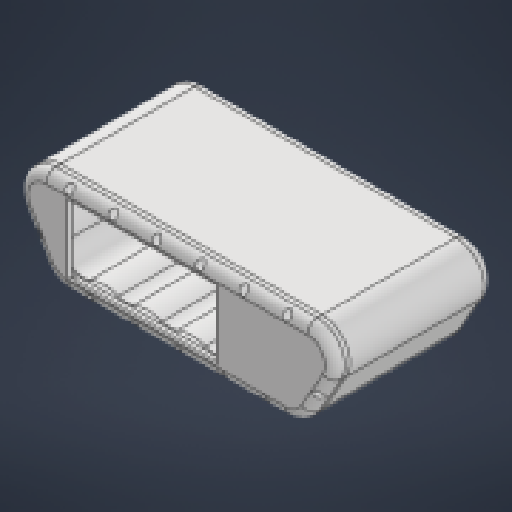
# Autodesk Inventor part: frame
Saved by Autodesk Inventor 2024 (Build 280153000, 153)
## iProperties
Created: 2024-05-04
Part Number: frame
Material: Generic
Document SubType Name: Modeling
Designer: markm
Density: 1 g/cm^3
Appearance: Default
Author: markm
Autodesk Inventor part; units mm, degrees
ref_plane "YZ Plane" through (0, 0, 0) normal (1, 0, 0) x (0, 1, 0)
ref_plane "XZ Plane" through (0, 0, 0) normal (0, 1, 0) x (-1, 0, 0)
ref_plane "XY Plane" through (0, 0, 0) normal (0, 0, 1) x (1, 0, 0)
sketch "Sketch1" plane through (0, 0, 0) normal (0, 0, 1) x (1, 0, 0)
  line L0 (0, -30.8093) -> (0, 30.8093) construction
  line L1 (78.1244, 2.5263) -> (67.1244, -16.5263)
  line L2 (55, -23.5263) -> (-55, -23.5263)
  line L3 (-67.1244, -16.5263) -> (-78.1244, 2.5263)
  arc A0 (-66, 23.5263) -> (-78.1244, 2.5263) centre (-66, 9.5263) ccw
  arc A1 (78.1244, 2.5263) -> (66, 23.5263) centre (66, 9.5263) ccw
  line L4 (-66, 9.5263) -> (-55, -9.5263) construction
  line L5 (-55, -9.5263) -> (55, -9.5263) construction
  line L6 (55, -9.5263) -> (66, 9.5263) construction
  line L7 (66, 9.5263) -> (-66, 9.5263) construction
  circle A2 centre (-66, 9.5263) radius 11
  circle A3 centre (-55, -9.5263) radius 11
  circle A4 centre (66, 9.5263) radius 11
  line L8 (-60.5, 0) -> (60.5, 0) construction
  circle A5 centre (-44, 9.5263) radius 11
  circle A6 centre (-33, -9.5263) radius 11
  circle A7 centre (-22, 9.5263) radius 11
  circle A8 centre (-11, -9.5263) radius 11
  circle A9 centre (0, 9.5263) radius 11
  circle A10 centre (11, -9.5263) radius 11
  circle A11 centre (22, 9.5263) radius 11
  circle A12 centre (33, -9.5263) radius 11
  circle A13 centre (44, 9.5263) radius 11
  circle A14 centre (55, -9.5263) radius 11
  arc A15 (-67.1244, -16.5263) -> (-55, -23.5263) centre (-55, -9.5263) ccw
  arc A16 (55, -23.5263) -> (67.1244, -16.5263) centre (55, -9.5263) ccw
  line L9 (-66, 23.5263) -> (66, 23.5263)
  arc A17 (75.9593, 3.7763) -> (66, 21.0263) centre (66, 9.5263) ccw construction
  line L10 (75.9593, 3.7763) -> (64.9593, -15.2763) construction
  arc A18 (55, -21.0263) -> (64.9593, -15.2763) centre (55, -9.5263) ccw construction
  line L11 (55, -21.0263) -> (-55, -21.0263) construction
  arc A19 (-64.9593, -15.2763) -> (-55, -21.0263) centre (-55, -9.5263) ccw construction
  line L12 (-64.9593, -15.2763) -> (-75.9593, 3.7763) construction
  arc A20 (-66, 21.0263) -> (-75.9593, 3.7763) centre (-66, 9.5263) ccw construction
  line L13 (-66, 21.0263) -> (66, 21.0263) construction
  arc A21 (72.9412, 0.9928) -> (65.8608, -11.2708) centre (85.4801, -14.4223) ccw
  line L14 (66, 9.5263) -> (33, -9.5263) construction
  line L15 (55, -9.5263) -> (44, 9.5263) construction
  arc A22 (47.9196, 19.8043) -> (62.0804, 19.8043) centre (55, 38.3708) ccw
  arc A23 (51.0804, -19.8043) -> (36.9196, -19.8043) centre (44, -38.3708) ccw
  line L16 (85.4801, -14.4223) -> (70.4593, -5.75) construction
  line L17 (55, 18.5) -> (55, 21.0263) construction
  line L18 (44, -18.5) -> (44, -21.0263) construction
  arc A24 (25.9196, 19.8043) -> (40.0804, 19.8043) centre (33, 38.3708) ccw
  line L19 (33, 18.5) -> (33, 21.0263) construction
  line L20 (22, -18.5) -> (22, -21.0263) construction
  arc A25 (29.0804, -19.8043) -> (14.9196, -19.8043) centre (22, -38.3708) ccw
  arc A26 (3.9196, 19.8043) -> (18.0804, 19.8043) centre (11, 38.3708) ccw
  line L21 (11, 18.5) -> (11, 21.0263) construction
  line L22 (0, -18.5) -> (0, -21.0263) construction
  arc A27 (7.0804, -19.8043) -> (-7.0804, -19.8043) centre (0, -38.3708) ccw
  arc A28 (-18.0804, 19.8043) -> (-3.9196, 19.8043) centre (-11, 38.3708) ccw
  line L23 (-11, 18.5) -> (-11, 21.0263) construction
  line L24 (-22, -18.5) -> (-22, -21.0263) construction
  arc A29 (-14.9196, -19.8043) -> (-29.0804, -19.8043) centre (-22, -38.3708) ccw
  arc A30 (-40.0804, 19.8043) -> (-25.9196, 19.8043) centre (-33, 38.3708) ccw
  line L25 (-33, 18.5) -> (-33, 21.0263) construction
  line L26 (-44, -18.5) -> (-44, -21.0263) construction
  arc A31 (-36.9196, -19.8043) -> (-51.0804, -19.8043) centre (-44, -38.3708) ccw
  arc A32 (-65.8608, -11.2708) -> (-72.9412, 0.9928) centre (-85.4801, -14.4223) ccw
  arc A33 (-62.0804, 19.8043) -> (-47.9196, 19.8043) centre (-55, 38.3708) ccw
  line L27 (-85.4801, -14.4223) -> (-70.4593, -5.75) construction
  line L28 (-55, 18.5) -> (-55, 21.0263) construction
  point P0 (0, 0)
  point P1 (0, 0)
  point P2 (44, -9.5263)
  point P3 (22, -9.5263)
  point P4 (0, -9.5263)
  point P5 (-22, -9.5263)
  point P6 (-44, -9.5263)
  point P7 (-60.5, 0)
  point P8 (-55, 9.5263)
  point P9 (-33, 9.5263)
  point P10 (-11, 9.5263)
  point P11 (11, 9.5263)
  point P12 (33, 9.5263)
  point P13 (55, 9.5263)
  point P14 (60.5, 0)
  point P15 (80, 9.5263)
  point P16 (47.9196, 19.8043)
  point P17 (62.0804, 19.8043)
  point P18 (51.0804, -19.8043)
  point P19 (36.9196, -19.8043)
  point P20 (-49.5, 0)
  point P21 (-38.5, 0)
  point P22 (-27.5, 0)
  point P23 (-16.5, 0)
  point P24 (-5.5, 0)
  point P25 (5.5, 0)
  point P26 (16.5, 0)
  point P27 (27.5, 0)
  point P28 (38.5, 0)
  point P29 (49.5, 0)
  point P30 (-62.0804, 19.8043)
  point P31 (-47.9196, 19.8043)
  point P32 (-40.0804, 19.8043)
  point P33 (-25.9196, 19.8043)
  point P34 (-18.0804, 19.8043)
  point P35 (-3.9196, 19.8043)
  point P36 (3.9196, 19.8043)
  point P37 (18.0804, 19.8043)
  point P38 (25.9196, 19.8043)
  point P39 (40.0804, 19.8043)
  point P40 (29.0804, -19.8043)
  point P41 (14.9196, -19.8043)
  point P42 (7.0804, -19.8043)
  point P43 (-7.0804, -19.8043)
  point P44 (-14.9196, -19.8043)
  point P45 (-29.0804, -19.8043)
  point P46 (-36.9196, -19.8043)
  point P47 (-51.0804, -19.8043)
  point P48 (-65.8608, -11.2708)
  point P49 (-72.9412, 0.9928)
  dimension "d70" = 22
  dimension "d73" = 22
  dimension "d106" = 14
  dimension "d122" = 14
  dimension "d174" = 2.5
  dimension "d182" = 37
  dimension "d185" = 22
  constraints: 59 end point, 45 point on circle, 32 centre point, 15 symmetric about line, 7 tangent, 5 coincident, 5 horizontal, 5 midpoint, 3 equal radius, 2 perpendicular, 2 point on line, 1 parallel, 101 other
  measures "d70" diameter of A2
  measures "d73" distance of A2.centre A5.centre
  measures "d106" radius of A16
  measures "d122" distance between parallel lines of L2 L5
  measures "d174" distance between parallel lines of L9 L13
  measures "d182" vertical distance of L18.start L17.start
  measures "d185" distance of A22.centre A24.centre
extrude "Extrusion1" add sketch "Sketch1" along normal mid plane 65
sketch "Sketch16" plane through (0, 0, -32.5) normal (0, 0, -1) x (-1, 0, 0)
  line L0 (67.1244, -16.5263) -> (78.1244, 2.5263) projected
  arc A0 (78.1244, 2.5263) -> (66, 23.5263) centre (66, 9.5263) ccw projected
  line L1 (66, 23.5263) -> (-66, 23.5263) projected
  arc A1 (-66, 23.5263) -> (-78.1244, 2.5263) centre (-66, 9.5263) ccw projected
  line L2 (-78.1244, 2.5263) -> (-67.1244, -16.5263) projected
  arc A2 (-67.1244, -16.5263) -> (-55, -23.5263) centre (-55, -9.5263) ccw projected
  line L3 (-55, -23.5263) -> (55, -23.5263) projected
  arc A3 (55, -23.5263) -> (67.1244, -16.5263) centre (55, -9.5263) ccw projected
  arc A4 (47.9196, 19.8043) -> (62.0804, 19.8043) centre (55, 38.3708) ccw projected
  arc A5 (72.9412, 0.9928) -> (62.0804, 19.8043) centre (66, 9.5263) ccw projected
  arc A6 (72.9412, 0.9928) -> (65.8608, -11.2708) centre (85.4801, -14.4223) ccw projected
  arc A7 (51.0804, -19.8043) -> (65.8608, -11.2708) centre (55, -9.5263) ccw projected
  arc A8 (51.0804, -19.8043) -> (36.9196, -19.8043) centre (44, -38.3708) ccw projected
  arc A9 (29.0804, -19.8043) -> (36.9196, -19.8043) centre (33, -9.5263) ccw projected
  arc A10 (29.0804, -19.8043) -> (14.9196, -19.8043) centre (22, -38.3708) ccw projected
  arc A11 (7.0804, -19.8043) -> (14.9196, -19.8043) centre (11, -9.5263) ccw projected
  arc A12 (7.0804, -19.8043) -> (-7.0804, -19.8043) centre (0, -38.3708) ccw projected
  arc A13 (-14.9196, -19.8043) -> (-7.0804, -19.8043) centre (-11, -9.5263) ccw projected
  arc A14 (-14.9196, -19.8043) -> (-29.0804, -19.8043) centre (-22, -38.3708) ccw projected
  arc A15 (-36.9196, -19.8043) -> (-29.0804, -19.8043) centre (-33, -9.5263) ccw projected
  arc A16 (-36.9196, -19.8043) -> (-51.0804, -19.8043) centre (-44, -38.3708) ccw projected
  arc A17 (-65.8608, -11.2708) -> (-51.0804, -19.8043) centre (-55, -9.5263) ccw projected
  arc A18 (-65.8608, -11.2708) -> (-72.9412, 0.9928) centre (-85.4801, -14.4223) ccw projected
  arc A19 (-62.0804, 19.8043) -> (-72.9412, 0.9928) centre (-66, 9.5263) ccw projected
  arc A20 (-62.0804, 19.8043) -> (-47.9196, 19.8043) centre (-55, 38.3708) ccw projected
  arc A21 (-40.0804, 19.8043) -> (-47.9196, 19.8043) centre (-44, 9.5263) ccw projected
  arc A22 (-40.0804, 19.8043) -> (-25.9196, 19.8043) centre (-33, 38.3708) ccw projected
  arc A23 (-18.0804, 19.8043) -> (-25.9196, 19.8043) centre (-22, 9.5263) ccw projected
  arc A24 (-18.0804, 19.8043) -> (-3.9196, 19.8043) centre (-11, 38.3708) ccw projected
  arc A25 (3.9196, 19.8043) -> (-3.9196, 19.8043) centre (0, 9.5263) ccw projected
  arc A26 (3.9196, 19.8043) -> (18.0804, 19.8043) centre (11, 38.3708) ccw projected
  arc A27 (25.9196, 19.8043) -> (18.0804, 19.8043) centre (22, 9.5263) ccw projected
  arc A28 (25.9196, 19.8043) -> (40.0804, 19.8043) centre (33, 38.3708) ccw projected
  arc A29 (47.9196, 19.8043) -> (40.0804, 19.8043) centre (44, 9.5263) ccw projected
  line L4 (-66, 18.5) -> (66, 18.5)
  arc A30 (73.7715, 5.0394) -> (66, 18.5) centre (66, 9.5263) ccw
  line L5 (73.7715, 5.0394) -> (62.7715, -14.0131)
  arc A31 (55, -18.5) -> (62.7715, -14.0131) centre (55, -9.5263) ccw
  line L6 (55, -18.5) -> (-55, -18.5)
  arc A32 (-62.7715, -14.0131) -> (-55, -18.5) centre (-55, -9.5263) ccw
  line L7 (-62.7715, -14.0131) -> (-73.7715, 5.0394)
  arc A33 (-66, 18.5) -> (-73.7715, 5.0394) centre (-66, 9.5263) ccw
  point P0 (0, 0)
  constraints: 8 end point, 8 point on circle, 4 centre point, 1 tangent, 7 other
extrude "Extrusion14" add sketch "Sketch16" along normal blind 7.5 contours A3 L3 A2 L2 A1 L1 A0 L0 | A4 L4 A28 A29 | L4 A30 L5 A31 L6 A32 L7 A33 | A4 A5 A6 L5 A30 L4 | L4 A26 A27 A28 | L4 A24 A25 A26 | A6 A7 A8 L6 A31 L5 | L4 A22 A23 A24 | L4 A20 A21 A22 | L4 A33 L7 A18 A19 A20 | A8 A9 A10 L6 | A10 A11 A12 L6 | A12 A13 A14 L6 | L7 A32 L6 A16 A17 A18 | A14 A15 A16 L6
extrude "Extrusion16" cut sketch "Sketch16" along normal blind 2.5 contours A4 L4 A28 A29 | L4 A30 L5 A31 L6 A32 L7 A33 | A4 A5 A6 L5 A30 L4 | L4 A26 A27 A28 | L4 A24 A25 A26 | A6 A7 A8 L6 A31 L5 | L4 A22 A23 A24 | L4 A20 A21 A22 | L4 A33 L7 A18 A19 A20 | A8 A9 A10 L6 | A10 A11 A12 L6 | A12 A13 A14 L6 | L7 A32 L6 A16 A17 A18 | A14 A15 A16 L6
extrude "Extrusion15" cut sketch "Sketch16" along normal blind 5 contours L4 A30 L5 A31 L6 A32 L7 A33
fillet "Fillet6" radius 5 8 edges at (78.1244, 16.5263, -40) (72.6244, -7, -40) (62, -21.6506, -40) (0, -23.5263, -40) (-62, -21.6506, -40) (-72.6244, -7, -40) (-78.1244, 16.5263, -40) (0, 23.5263, -40)
sketch "Sketch20" plane through (0, 0, 32.5) normal (0, 0, 1) x (1, 0, 0)
  line L0 (-78.1244, 2.5263) -> (-67.1244, -16.5263) projected
  arc A0 (-67.1244, -16.5263) -> (-55, -23.5263) centre (-55, -9.5263) ccw projected
  line L1 (-55, -23.5263) -> (55, -23.5263) projected
  arc A1 (55, -23.5263) -> (67.1244, -16.5263) centre (55, -9.5263) ccw projected
  line L2 (67.1244, -16.5263) -> (78.1244, 2.5263) projected
  arc A2 (78.1244, 2.5263) -> (66, 23.5263) centre (66, 9.5263) ccw projected
  line L3 (66, 23.5263) -> (-66, 23.5263) projected
  arc A3 (-66, 23.5263) -> (-78.1244, 2.5263) centre (-66, 9.5263) ccw projected
  arc A4 (-62.0804, 19.8043) -> (-47.9196, 19.8043) centre (-55, 38.3708) ccw projected
  arc A5 (-40.0804, 19.8043) -> (-47.9196, 19.8043) centre (-44, 9.5263) ccw projected
  arc A6 (-40.0804, 19.8043) -> (-25.9196, 19.8043) centre (-33, 38.3708) ccw projected
  arc A7 (-18.0804, 19.8043) -> (-25.9196, 19.8043) centre (-22, 9.5263) ccw projected
  arc A8 (-18.0804, 19.8043) -> (-3.9196, 19.8043) centre (-11, 38.3708) ccw projected
  arc A9 (3.9196, 19.8043) -> (-3.9196, 19.8043) centre (0, 9.5263) ccw projected
  arc A10 (3.9196, 19.8043) -> (18.0804, 19.8043) centre (11, 38.3708) ccw projected
  arc A11 (25.9196, 19.8043) -> (18.0804, 19.8043) centre (22, 9.5263) ccw projected
  arc A12 (25.9196, 19.8043) -> (40.0804, 19.8043) centre (33, 38.3708) ccw projected
  arc A13 (47.9196, 19.8043) -> (40.0804, 19.8043) centre (44, 9.5263) ccw projected
  arc A14 (47.9196, 19.8043) -> (62.0804, 19.8043) centre (55, 38.3708) ccw projected
  arc A15 (72.9412, 0.9928) -> (62.0804, 19.8043) centre (66, 9.5263) ccw projected
  arc A16 (72.9412, 0.9928) -> (65.8608, -11.2708) centre (85.4801, -14.4223) ccw projected
  arc A17 (51.0804, -19.8043) -> (65.8608, -11.2708) centre (55, -9.5263) ccw projected
  arc A18 (51.0804, -19.8043) -> (36.9196, -19.8043) centre (44, -38.3708) ccw projected
  arc A19 (29.0804, -19.8043) -> (36.9196, -19.8043) centre (33, -9.5263) ccw projected
  arc A20 (29.0804, -19.8043) -> (14.9196, -19.8043) centre (22, -38.3708) ccw projected
  arc A21 (7.0804, -19.8043) -> (14.9196, -19.8043) centre (11, -9.5263) ccw projected
  arc A22 (7.0804, -19.8043) -> (-7.0804, -19.8043) centre (0, -38.3708) ccw projected
  arc A23 (-14.9196, -19.8043) -> (-7.0804, -19.8043) centre (-11, -9.5263) ccw projected
  arc A24 (-14.9196, -19.8043) -> (-29.0804, -19.8043) centre (-22, -38.3708) ccw projected
  arc A25 (-36.9196, -19.8043) -> (-29.0804, -19.8043) centre (-33, -9.5263) ccw projected
  arc A26 (-36.9196, -19.8043) -> (-51.0804, -19.8043) centre (-44, -38.3708) ccw projected
  arc A27 (-65.8608, -11.2708) -> (-51.0804, -19.8043) centre (-55, -9.5263) ccw projected
  arc A28 (-65.8608, -11.2708) -> (-72.9412, 0.9928) centre (-85.4801, -14.4223) ccw projected
  arc A29 (-62.0804, 19.8043) -> (-72.9412, 0.9928) centre (-66, 9.5263) ccw projected
  line L4 (-66, 18.5) -> (66, 18.5)
  arc A30 (73.7715, 5.0394) -> (66, 18.5) centre (66, 9.5263) ccw
  line L5 (73.7715, 5.0394) -> (62.7715, -14.0131)
  arc A31 (55, -18.5) -> (62.7715, -14.0131) centre (55, -9.5263) ccw
  line L6 (55, -18.5) -> (-55, -18.5)
  arc A32 (-62.7715, -14.0131) -> (-55, -18.5) centre (-55, -9.5263) ccw
  line L7 (-62.7715, -14.0131) -> (-73.7715, 5.0394)
  arc A33 (-66, 18.5) -> (-73.7715, 5.0394) centre (-66, 9.5263) ccw
  arc A34 (-65.8608, -11.2708) -> (-72.9412, 0.9928) centre (-85.4801, -14.4223) ccw projected
  point P0 (0, 0)
  constraints: 8 end point, 8 point on circle, 4 centre point, 1 tangent, 7 other
extrude "Extrusion17" add sketch "Sketch20" along normal blind 7.5 separate body contours A3 L3 A2 L2 A1 L1 A0 L0 | A4 L4 A33 L7 A28 A29 | L4 A30 L5 A31 L6 A32 L7 A33 | A4 A5 A6 L4 | A6 A7 A8 L4 | L7 A32 L6 A26 A27 A28 | A8 A9 A10 L4 | A10 A11 A12 L4 | A12 A13 A14 L4 | L6 A24 A25 A26 | A14 A15 A16 L5 A30 L4 | L6 A22 A23 A24 | L6 A20 A21 A22 | L6 A18 A19 A20 | A16 A17 A18 L6 A31 L5
extrude "Extrusion18" cut sketch "Sketch20" along normal blind 2.75 contours A4 L4 A33 L7 A28 A29 | L4 A30 L5 A31 L6 A32 L7 A33 | A4 A5 A6 L4 | A6 A7 A8 L4 | L7 A32 L6 A26 A27 A28 | A8 A9 A10 L4 | A10 A11 A12 L4 | A12 A13 A14 L4 | L6 A24 A25 A26 | A14 A15 A16 L5 A30 L4 | L6 A22 A23 A24 | L6 A20 A21 A22 | L6 A18 A19 A20 | A16 A17 A18 L6 A31 L5 bodies 1 2
extrude "Extrusion19" cut sketch "Sketch20" along normal blind 5 contours L4 A30 L5 A31 L6 A32 L7 A33 bodies 1 2
fillet "Fillet7" radius 5 8 edges at (0, 23.5263, 40) (-78.1244, 16.5263, 40) (-72.6244, -7, 40) (-62, -21.6506, 40) (0, -23.5263, 40) (62, -21.6506, 40) (72.6244, -7, 40) (78.1244, 16.5263, 40)
sketch "Sketch18" plane through (0, 0, 40) normal (0, 0, 1) x (1, 0, 0)
  point P0 (0, 0)
  point P1 (-55, 21.0263)
  point P2 (-33, 21.0263)
  point P3 (-11, 21.0263)
  point P4 (11, 21.0263)
  point P5 (33, 21.0263)
  point P6 (55, 21.0263)
  point P7 (70.4593, -5.75)
  point P8 (44, -21.0263)
  point P9 (22, -21.0263)
  point P10 (0, -21.0263)
  point P11 (-22, -21.0263)
  point P12 (-44, -21.0263)
  point P13 (-70.4593, -5.75)
hole "Hole4" at (-55, 21.0263, 40) at (-33, 21.0263, 40) at (-11, 21.0263, 40) at (11, 21.0263, 40) at (33, 21.0263, 40) at (55, 21.0263, 40) at (70.4593, -5.75, 40) at (44, -21.0263, 40) at (22, -21.0263, 40) at (0, -21.0263, 40) at (-22, -21.0263, 40) at (-44, -21.0263, 40) at (-70.4593, -5.75, 40) direction (0, 0, -1) diameter 2.2 depth 15 counterbore diameter 4 counterbore depth 5 bodies 1 2
sketch "Sketch26" plane through (0, 0, 37.5) normal (0, 0, -1) x (-1, 0, 0)
  line L0 (55, -18.5) -> (-55, -18.5) projected
  arc A0 (55, -18.5) -> (62.7715, -14.0131) centre (55, -9.5263) ccw projected
  line L1 (73.7715, 5.0394) -> (62.7715, -14.0131) projected
  arc A1 (73.7715, 5.0394) -> (66, 18.5) centre (66, 9.5263) ccw projected
  line L2 (-66, 18.5) -> (66, 18.5) projected
  arc A2 (-66, 18.5) -> (-73.7715, 5.0394) centre (-66, 9.5263) ccw projected
  line L3 (-62.7715, -14.0131) -> (-73.7715, 5.0394) projected
  arc A3 (-62.7715, -14.0131) -> (-55, -18.5) centre (-55, -9.5263) ccw projected
  arc A4 (72.9054, 5.5394) -> (66, 17.5) centre (66, 9.5263) ccw
  line L4 (72.9054, 5.5394) -> (61.9054, -13.5131)
  arc A5 (55, -17.5) -> (61.9054, -13.5131) centre (55, -9.5263) ccw
  line L5 (55, -17.5) -> (-55, -17.5)
  arc A6 (-61.9054, -13.5131) -> (-55, -17.5) centre (-55, -9.5263) ccw
  line L6 (-61.9054, -13.5131) -> (-72.9054, 5.5394)
  arc A7 (-66, 17.5) -> (-72.9054, 5.5394) centre (-66, 9.5263) ccw
  line L7 (-66, 17.5) -> (66, 17.5)
  line L8 (55, -18.5) -> (55, 18.5)
  line L9 (-20, 18.5) -> (-20, -18.5)
  point P0 (0, 0)
  point P1 (-20, 17.5)
  point P2 (-20, -17.5)
  point P3 (55, -17.5)
  point P4 (55, 17.5)
  dimension "d259" = 1
  dimension "d295" = 75
  constraints: 12 end point, 8 point on circle, 4 centre point, 3 point on line, 2 perpendicular, 7 other
  measures "d259" distance between parallel lines of L2 L7
  measures "d295" distance between parallel lines of L9 L8
extrude "Extrusion23" cut sketch "Sketch26" against normal through all contours L5 L9 L7 L8 bodies 2
chamfer "Chamfer10" distance 1 distance2 2.5 2 edges at (-17.5, -17.5, 37.5) (-17.5, 17.5, 37.5) measured on face at (-17.5, -18, 37.5) measured on face at (-17.5, 18, 37.5)
sketch "Sketch29" plane through (0, 0, 37.5) normal (0, 0, -1) x (-1, 0, 0)
  line L0 (-20, 17.5) -> (-20, -17.5) projected
  line L1 (-20, 2.5) -> (-47.4904, 2.5)
  line L2 (-47.4904, -2.5) -> (-20, -2.5)
  line L3 (0, 0) -> (-49.5, 0) construction
  line L4 (-49.5, 0) -> (-60.2935, 6.2316) construction
  line L5 (-49.9904, 3.1699) -> (-64.75, 11.6913)
  line L6 (-69.8322, 8.8521) -> (-52.4904, -1.1603)
  arc A0 (-62.0804, 19.8043) -> (-72.9412, 0.9928) centre (-66, 9.5263) ccw projected
  arc A1 (-49.9904, 3.1699) -> (-47.4904, 2.5) centre (-47.4904, 7.5) ccw
  arc A2 (-52.4904, -1.1603) -> (-47.4904, -2.5) centre (-47.4904, 7.5) ccw
  arc A3 (-64.75, 11.6913) -> (-67.25, 7.3612) centre (-66, 9.5263) ccw
  point P0 (-62.7599, 0)
  point P1 (-62.7599, 0)
  dimension "d304" = 5
  dimension "d307" = 30
  dimension "d308" = 5
  dimension "d309" = 5
  constraints: 12 end point, 6 point on circle, 5 tangent, 4 horizontal, 4 point on line, 3 centre point, 2 coincident, 2 parallel, 1 concentric, 3 other
  measures "d304" distance between parallel lines of L2 L1
  measures "d307" angle of L3 L4
  measures "d308" distance of L5.end A3.end
  measures "d309" radius of A1
extrude "Extrusion25" cut sketch "Sketch29" against normal blind 2 bodies 2
fillet "Fillet9" radius 1 6 edges at (48.7845, 2.6704, 39.5) (57.3702, 7.4306, 39.5) (59.8702, 3.1005, 39.5) (50.0786, -2.1593, 39.5) (33.7452, -2.5, 39.5) (33.7452, 2.5, 39.5)
thicken "Thicken11" operation cut thickness 0.25 both sides no extend neighbours yes toward (-1, 0, 0) bodies 2 faces at (-55, -5.8333, 38.3333) (20, 12.8333, 38.3333)
body "Solid1"
body "Solid5"
